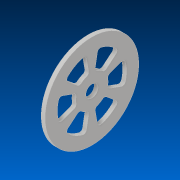
# Autodesk Inventor part: paddlewheel_outer
Saved by Autodesk Inventor 2019 (Build 230136000, 136)
## iProperties
Created: 2018-08-23
Part Number: paddlewheel_outer
Material: Generic
Document SubType Name: Modeling
Designer: Kitte_X
Density: 1 g/cm^3
Appearance: Default
Author: Kitte_X
Autodesk Inventor part; units mm, degrees
ref_plane "YZ Plane" through (0, 0, 0) normal (1, 0, 0) x (0, 1, 0)
ref_plane "XZ Plane" through (0, 0, 0) normal (0, 1, 0) x (-1, 0, 0)
ref_plane "XY Plane" through (0, 0, 0) normal (0, 0, 1) x (1, 0, 0)
sketch "Sketch1" plane through (0, 0, 0) normal (1, 0, 0) x (0, 1, 0)
  circle A0 centre (0, 0) radius 76.2
  line L0 (0, 0) -> (44.7892, 61.6471) construction
  line L1 (0, 0) -> (-44.7892, 61.6471) construction
  line L2 (0, 0) -> (-26.0619, 71.6046) construction
  line L3 (0, -76.2) -> (0, 76.2) construction
  line L4 (-10.5331, 28.9395) -> (-17.4277, 47.8823)
  arc A1 (13.9724, 54.4354) -> (-13.9724, 54.4354) centre (0, 0) ccw
  arc A2 (4.8996, 25.7378) -> (-4.8996, 25.7378) centre (0, 0) ccw
  arc A3 (17.4277, 47.8823) -> (13.9724, 54.4354) centre (12.7293, 49.5924) ccw
  arc A4 (4.8996, 25.7378) -> (10.5331, 28.9395) centre (5.8346, 30.6496) ccw
  arc A5 (-10.5331, 28.9395) -> (-4.8996, 25.7378) centre (-5.8346, 30.6496) ccw
  arc A6 (-13.9724, 54.4354) -> (-17.4277, 47.8823) centre (-12.7293, 49.5924) ccw
  line L5 (0, 0) -> (26.0619, 71.6046) construction
  line L6 (17.4277, 47.8823) -> (10.5331, 28.9395)
  line L7 (-32.7534, 39.034) -> (-19.7958, 23.5917)
  arc A7 (-32.7534, 39.034) -> (-40.1563, 39.3181) centre (-36.5836, 35.8201) ccw
  arc A8 (-19.8398, 17.1121) -> (-19.7958, 23.5917) centre (-23.626, 20.3777) ccw
  line L8 (-30.3289, 5.3478) -> (-50.1811, 8.8483)
  arc A9 (-30.3289, 5.3478) -> (-24.7394, 8.6257) centre (-29.4606, 10.2718) ccw
  arc A10 (-19.8398, 17.1121) -> (-24.7394, 8.6257) centre (0, 0) ccw
  arc A11 (-40.1563, 39.3181) -> (-54.1286, 15.1173) centre (0, 0) ccw
  arc A12 (-54.1286, 15.1173) -> (-50.1811, 8.8483) centre (-49.3129, 13.7723) ccw
  line L9 (-50.1811, -8.8483) -> (-30.3289, -5.3478)
  arc A13 (-50.1811, -8.8483) -> (-54.1286, -15.1173) centre (-49.3129, -13.7723) ccw
  arc A14 (-24.7394, -8.6257) -> (-30.3289, -5.3478) centre (-29.4606, -10.2718) ccw
  line L10 (-19.7958, -23.5917) -> (-32.7534, -39.034)
  arc A15 (-19.7958, -23.5917) -> (-19.8398, -17.1121) centre (-23.626, -20.3777) ccw
  arc A16 (-24.7394, -8.6257) -> (-19.8398, -17.1121) centre (0, 0) ccw
  arc A17 (-54.1286, -15.1173) -> (-40.1563, -39.3181) centre (0, 0) ccw
  arc A18 (-40.1563, -39.3181) -> (-32.7534, -39.034) centre (-36.5836, -35.8201) ccw
  line L11 (-17.4277, -47.8823) -> (-10.5331, -28.9395)
  arc A19 (-17.4277, -47.8823) -> (-13.9724, -54.4354) centre (-12.7293, -49.5924) ccw
  arc A20 (-4.8996, -25.7378) -> (-10.5331, -28.9395) centre (-5.8346, -30.6496) ccw
  line L12 (10.5331, -28.9395) -> (17.4277, -47.8823)
  arc A21 (10.5331, -28.9395) -> (4.8996, -25.7378) centre (5.8346, -30.6496) ccw
  arc A22 (-4.8996, -25.7378) -> (4.8996, -25.7378) centre (0, 0) ccw
  arc A23 (-13.9724, -54.4354) -> (13.9724, -54.4354) centre (0, 0) ccw
  arc A24 (13.9724, -54.4354) -> (17.4277, -47.8823) centre (12.7293, -49.5924) ccw
  line L13 (32.7534, -39.034) -> (19.7958, -23.5917)
  arc A25 (32.7534, -39.034) -> (40.1563, -39.3181) centre (36.5836, -35.8201) ccw
  arc A26 (19.8398, -17.1121) -> (19.7958, -23.5917) centre (23.626, -20.3777) ccw
  line L14 (30.3289, -5.3478) -> (50.1811, -8.8483)
  arc A27 (30.3289, -5.3478) -> (24.7394, -8.6257) centre (29.4606, -10.2718) ccw
  arc A28 (19.8398, -17.1121) -> (24.7394, -8.6257) centre (0, 0) ccw
  arc A29 (40.1563, -39.3181) -> (54.1286, -15.1173) centre (0, 0) ccw
  arc A30 (54.1286, -15.1173) -> (50.1811, -8.8483) centre (49.3129, -13.7723) ccw
  circle A31 centre (0, 0) radius 10
  circle A32 centre (0, 0) radius 26.2 construction
  line L15 (50.1811, 8.8483) -> (30.3289, 5.3478)
  arc A33 (50.1811, 8.8483) -> (54.1286, 15.1173) centre (49.3129, 13.7723) ccw
  arc A34 (24.7394, 8.6257) -> (30.3289, 5.3478) centre (29.4606, 10.2718) ccw
  line L16 (19.7958, 23.5917) -> (32.7534, 39.034)
  arc A35 (19.7958, 23.5917) -> (19.8398, 17.1121) centre (23.626, 20.3777) ccw
  arc A36 (24.7394, 8.6257) -> (19.8398, 17.1121) centre (0, 0) ccw
  arc A37 (54.1286, 15.1173) -> (40.1563, 39.3181) centre (0, 0) ccw
  arc A38 (40.1563, 39.3181) -> (32.7534, 39.034) centre (36.5836, 35.8201) ccw
  point P0 (8.9609, 24.6199)
  point P1 (-8.9609, 24.6199)
  point P2 (-19.2215, 52.8107)
  dimension "d1" = 72
  dimension "d4" = 16
  dimension "d7" = 20
  dimension "d8" = 152.4
  dimension "d9" = 30
  dimension "d10" = 5
  dimension "d11" = 5
  dimension "d12" = 36
  dimension "d13" = 20
  dimension "d16" = 360
  dimension "d18" = 20
  dimension "d21" = 52.4
  constraints: 81 point on circle, 39 centre point, 34 end point, 7 concentric, 6 tangent, 4 point on line, 3 coincident, 2 equal radius, 1 collinear, 1 vertical, 133 other
  measures "d1" angle of L1 L0
  measures "d4" angle of L1 L2
  measures "d7" radial gap between concentric circles of A0 A1
  measures "d8" distance of L3.start L3.end
  measures "d9" radial gap between concentric circles of A1 A2
  measures "d10" radius of A3
  measures "d11" radius of A4
  measures "d12" angle of L0 L3
  measures "d13" angle of L3 L5
  measures "d18" diameter of A31
  measures "d21" diameter of A32
extrude "Extrusion2" add sketch "Sketch1" along normal blind 6.35
body "Solid2"
